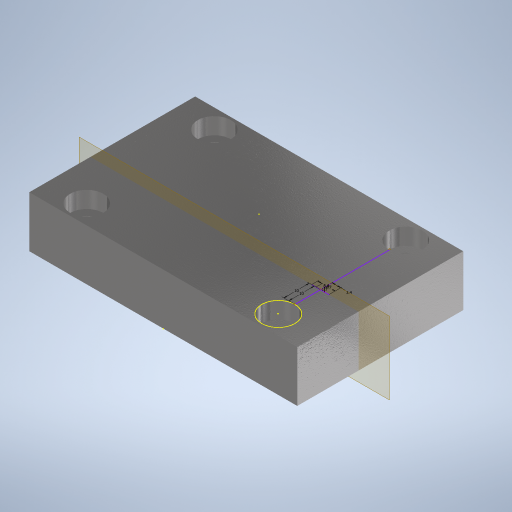
# Autodesk Inventor part: Soporte
Saved by Autodesk Inventor 2023 (Build 270158000, 158)
## iProperties
Created: 2018-04-04
Part Number: Soporte
Material: Generic
Document SubType Name: Modeling
Designer: Hogar
Density: 1 g/cm^3
Appearance: Galvanized
Author: Hogar
Autodesk Inventor part; units mm, degrees
ref_plane "YZ Plane" through (0, 0, 0) normal (1, 0, 0) x (0, 1, 0)
ref_plane "XZ Plane" through (0, 0, 0) normal (0, 1, 0) x (-1, 0, 0)
sketch "Sketch1" plane through (0, 0, 0) normal (0, 0, 1) x (1, 0, 0)
  line L0 (-52.5, -37.5) -> (52.5, -37.5)
  line L1 (52.5, -37.5) -> (52.5, 37.5)
  line L2 (52.5, 37.5) -> (-52.5, 37.5)
  line L3 (-52.5, 37.5) -> (-52.5, -37.5)
  line L4 (-52.5, -37.5) -> (52.5, 37.5) construction
  line L5 (52.5, -37.5) -> (-52.5, 37.5) construction
  point P0 (0, 0)
  dimension "d0" = 105
  dimension "d1" = 75
  constraints: 12 end point, 2 midpoint, 2 parallel, 1 horizontal, 1 perpendicular
  measures "d0" distance of L2.end L1.end
  measures "d1" distance of L1.end L0.end
extrude "Extrusion1" add sketch "Sketch1" along normal blind 20
sketch "Sketch2" plane through (0, 0, 20) normal (0, 0, 1) x (1, 0, 0)
  line L0 (52.5, 37.5) -> (-52.5, 37.5) projected
  line L1 (-52.5, 37.5) -> (-52.5, -37.5) projected
  point P0 (0, 0)
  point P1 (-37.5, 20)
  point P2 (37.5, 20)
  point P3 (-37.5, -30)
  point P4 (37.5, -30)
  dimension "d4" = 75
  dimension "d5" = 17.5
  dimension "d6" = 17.5
  dimension "d7" = 15
  dimension "d8" = 50
  dimension "d9" = 50
  dimension "d10" = 75
  dimension "d11" = 15
  measures "d4" distance of point (37.5, 20) point (-37.5, 20)
  measures "d5" distance from line of L0 point (-37.5, 20)
  measures "d6" distance from line of L0 point (37.5, 20)
  measures "d7" distance from line of L1 point (-37.5, 20)
  measures "d8" distance of point (-37.5, -30) point (-37.5, 20)
  measures "d9" distance of point (37.5, 20) point (37.5, -30)
  measures "d10" distance of point (37.5, -30) point (-37.5, -30)
  measures "d11" distance from line of L1 point (-37.5, -30)
hole "Hole1" at (-37.5, 20, 20) at (37.5, 20, 20) at (-37.5, -30, 20) at (37.5, -30, 20) direction (0, 0, -1) diameter 6.4 end through all counterbore diameter 13 counterbore depth 6.5 clearance for "Hex Head Bolt" size "M6" standard "Ansi Metric M Profile"
sketch "Sketch4" plane through (52.5, -37.5, 0) normal (1, 0, 0) x (0, 0, -1)
  line L0 (0, 75) -> (-20, 75) projected
  line L1 (-20, 75) -> (0, 75)
  line L2 (0, 75) -> (0, 65)
  line L3 (0, 65) -> (-20, 65)
  line L4 (-20, 65) -> (-20, 75)
  dimension "d19" = 20
  dimension "d20" = 10
  constraints: 8 end point, 2 parallel, 1 horizontal, 1 perpendicular
  measures "d19" distance of L2.end L3.end
  measures "d20" distance of L1.end L2.end
extrude "Extrusion2" cut sketch "Sketch4" against normal through all
sketch "Sketch5" plane through (-52.5, -37.5, 0) normal (0, -1, 0) x (1, 0, 0)
  point P0 (52.5, 0)
sketch "Sketch7" plane through (0, 0, 20) normal (0, 0, 1) x (1, 0, 0)
  line L0 (37.5265, 13.5317) -> (37.5265, -23.5001)
  circle A0 centre (37.5, -30) radius 6.5 projected
  line L1 (37.5265, -23.5001) -> (37.5265, -13.5001)
  line L2 (37.5265, -13.5001) -> (40.9265, -13.5001)
  line L3 (40.9265, -13.5001) -> (34.1265, -13.5001)
  line L4 (37.5265, -13.5001) -> (39.2265, -13.5001)
  line L5 (39.2265, -13.5001) -> (35.8265, -13.5001)
  point P0 (0, 0)
  dimension "d41" = 10
  dimension "d42" = 3.4
  dimension "d43" = 6.8
  dimension "d44" = 1.7
  dimension "d45" = 3.4
  constraints: 12 end point, 4 point on line, 1 perpendicular, 1 vertical, 2 other
  measures "d41" distance of L0.end L1.end
  measures "d42" distance of L1.end L2.end
  measures "d43" distance of L2.end L3.end
  measures "d44" distance of L1.end L4.end
  measures "d45" distance of L4.end L5.end
sketch "Sketch8" plane through (0, 0, 20) normal (0, 0, 1) x (1, 0, 0)
  circle A0 centre (37.5, -30) radius 6.5 projected
  line L0 (37.5, -23.5) -> (37.5, -13.5)
  point P0 (0, 0)
  dimension "d25" = 10
  constraints: 2 end point, 1 vertical, 1 vertical alignment, 1 other
  measures "d25" distance of L0.start L0.end
ref_plane "Work Plane3" through (37.5, -13.5, 20) normal (0, -1, 0) x (1, 0, 0)
ref_plane "Work Plane4" through (37.5265, -13.5001, 20) normal (0, -1, 0) x (1, 0, 0)
sketch "Sketch10" plane through (37.5265, -13.5001, 20) normal (0, -1, 0) x (1, 0, 0)
  line L0 (1.6997, -0.0003) -> (1.6997, 1.6997)
  line L1 (-1.7001, -0.0003) -> (-1.7001, 1.6997)
  point P0 (-37.5265, -20)
  dimension "d46" = 1.7
  dimension "d47" = 1.7
  constraints: 4 end point, 2 vertical
  measures "d46" distance of L0.start L0.end
  measures "d47" distance of L1.start L1.end
hole "Hole3" at (35.8265, -13.5001, 21.6997) direction (0, 1, 0) diameter 3 depth 17
sketch "Sketch12" plane through (37.5265, -13.5001, 20) normal (0, -1, 0) x (1, 0, 0)
  line L0 (1.6597, 0) -> (1.7401, 0) projected
  line L1 (1.6999, 0) -> (1.6999, 1.7)
  point P0 (-37.5265, -20)
  dimension "d59" = 1.7
  constraints: 2 end point, 1 midpoint, 1 vertical
  measures "d59" distance of L1.start L1.end
equation "\"d6\" = d5"
equation "\"d9\" = d8"
equation "\"d10\" = d4"
equation "\"d11\" = d7"
body "Solid1"
